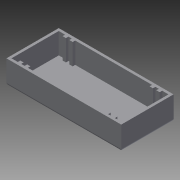
# Autodesk Inventor part: Unterteil
Saved by Autodesk Inventor 2015 (Build 190159000, 159)
## iProperties
Created: 2015-01-18
Part Number: Unterteil
Material: Generisch
Document SubType Name: Modeling
Designer: Jacob
Density: 1 g/cm^3
Appearance: Vorgabe
Author: Jacob
Autodesk Inventor part; units mm, degrees
ref_plane "YZ Plane" through (0, 0, 0) normal (1, 0, 0) x (0, 1, 0)
ref_plane "XZ Plane" through (0, 0, 0) normal (0, 1, 0) x (-1, 0, 0)
ref_plane "XY Plane" through (0, 0, 0) normal (0, 0, 1) x (1, 0, 0)
sketch "Skizze2" plane through (0, 0, 0) normal (0, 0, 1) x (1, 0, 0)
  line L0 (-32.5, 14) -> (32.5, 14)
  line L1 (32.5, 14) -> (32.5, -14)
  line L2 (32.5, -14) -> (-32.5, -14)
  line L3 (-32.5, -14) -> (-32.5, 14)
  line L4 (-32.5, 14) -> (32.5, -14) construction
  line L5 (32.5, 14) -> (-32.5, -14) construction
  point P0 (0, 0)
  dimension "d0" = 65
  dimension "d1" = 28
  constraints: 12 end point, 2 midpoint, 2 parallel, 1 horizontal, 1 perpendicular
  measures "d0" distance of L1.end L2.end
  measures "d1" distance of L0.end L1.end
extrude "Extrusion1" add sketch "Skizze2" along normal blind 1.5
sketch "Skizze4" plane through (0, 0, 0) normal (0, 0, -1) x (-1, 0, 0)
  line L0 (32.5, 14) -> (-32.5, 14) projected
  line L1 (-32.5, 14) -> (-32.5, -14) projected
  line L2 (-32.5, -14) -> (32.5, -14) projected
  line L3 (32.5, -14) -> (32.5, 14) projected
  line L4 (34, -15.5) -> (-34, -15.5)
  line L5 (-34, -15.5) -> (-34, 15.5)
  line L6 (-34, 15.5) -> (34, 15.5)
  line L7 (34, 15.5) -> (34, -15.5)
  point P0 (0, 0)
  dimension "d4" = 1.5
  constraints: 8 end point, 3 other
  measures "d4" distance between parallel lines of L2 L4
extrude "Extrusion2" add sketch "Skizze4" against normal blind 14
fillet "Rundung1" radius 1.5 4 edges at (0, -15.5, 0) (0, 15.5, 0) (34, 0, 0) (-34, 0, 0)
sketch "Skizze5" plane through (0, 0, 1.5) normal (0, 0, 1) x (1, 0, 0)
  line L0 (0, -21.0221) -> (0, 21.9802) construction
  line L1 (-32.5, -14) -> (32.5, -14) projected
  line L2 (-28.7599, -14) -> (-26.7599, -14)
  line L3 (-26.7599, -14) -> (-26.7599, -12.5)
  line L4 (-26.7599, -12.5) -> (-28.7599, -12.5)
  line L5 (-28.7599, -12.5) -> (-28.7599, -14)
  line L6 (-24.7599, -14) -> (-22.7599, -14)
  line L7 (-22.7599, -14) -> (-22.7599, -12.5)
  line L8 (-22.7599, -12.5) -> (-24.7599, -12.5)
  line L9 (-24.7599, -12.5) -> (-24.7599, -14)
  line L10 (-34, 15.5) -> (-34, -15.5) construction
  line L11 (-34, 0) -> (34, 0) construction
  line L12 (34, -15.5) -> (34, 15.5) construction
  line L13 (28.7599, -14) -> (26.7599, -14)
  line L14 (26.7599, -14) -> (26.7599, -12.5)
  line L15 (26.7599, -12.5) -> (28.7599, -12.5)
  line L16 (28.7599, -12.5) -> (28.7599, -14)
  line L17 (24.7599, -14) -> (22.7599, -14)
  line L18 (22.7599, -14) -> (22.7599, -12.5)
  line L19 (22.7599, -12.5) -> (24.7599, -12.5)
  line L20 (24.7599, -12.5) -> (24.7599, -14)
  line L21 (34, 15.5) -> (34, -15.5) construction
  line L22 (-28.7599, 14) -> (-26.7599, 14)
  line L23 (-26.7599, 14) -> (-26.7599, 12.5)
  line L24 (-26.7599, 12.5) -> (-28.7599, 12.5)
  line L25 (-28.7599, 12.5) -> (-28.7599, 14)
  line L26 (-24.7599, 14) -> (-22.7599, 14)
  line L27 (-22.7599, 14) -> (-22.7599, 12.5)
  line L28 (-22.7599, 12.5) -> (-24.7599, 12.5)
  line L29 (-24.7599, 12.5) -> (-24.7599, 14)
  line L30 (22.7599, 14) -> (22.7599, 12.5)
  line L31 (24.7599, 14) -> (22.7599, 14)
  line L32 (22.7599, 12.5) -> (24.7599, 12.5)
  line L33 (24.7599, 12.5) -> (24.7599, 14)
  line L34 (26.7599, 14) -> (26.7599, 12.5)
  line L35 (28.7599, 14) -> (26.7599, 14)
  line L36 (26.7599, 12.5) -> (28.7599, 12.5)
  line L37 (28.7599, 12.5) -> (28.7599, 14)
  point P0 (0, 0)
  dimension "d11" = 2
  dimension "d12" = 1.5
  dimension "d13" = 2
  dimension "d14" = 2
  constraints: 70 end point, 24 symmetric about line, 6 point on line, 4 parallel, 2 horizontal, 2 midpoint, 2 perpendicular, 1 vertical
  measures "d11" distance of L4.end L3.end
  measures "d12" distance of L3.end L2.end
  measures "d13" distance of L8.end L7.end
  measures "d14" distance between parallel lines of L9 L3
extrude "Extrusion4" add sketch "Skizze5" along normal blind 12.5
